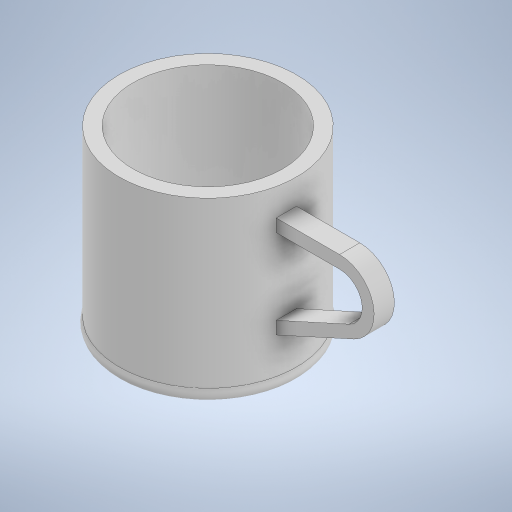
# Autodesk Inventor part: TAZA DEL CID
Saved by Autodesk Inventor 2024 (Build 280153000, 153)
## iProperties
Created: 2024-02-22
Part Number: TAZA DEL CID
Material: Genérico
Document SubType Name: Modeling
Designer: fenyc
Density: 1 g/cm^3
Appearance: Valor por defecto
Author: fenyc
Autodesk Inventor part; units mm, degrees
ref_plane "YZ Plane" through (0, 0, 0) normal (1, 0, 0) x (0, 1, 0)
ref_plane "XZ Plane" through (0, 0, 0) normal (0, 1, 0) x (-1, 0, 0)
ref_plane "XY Plane" through (0, 0, 0) normal (0, 0, 1) x (1, 0, 0)
sketch "Boceto1" plane through (0, 0, 0) normal (0, 0, 1) x (1, 0, 0)
  line L0 (-26.211, 0) -> (6.289, 0)
  line L1 (6.289, 0) -> (6.289, 70)
  line L2 (6.289, 70) -> (-28.711, 70)
  line L3 (-28.711, 70) -> (-28.711, 5)
  arc A0 (-28.711, 5) -> (-26.211, 0) centre (-26.211, 3.125) ccw
  point P0 (0, 0)
  dimension "d2" = 32.5
  dimension "d3" = 70
  dimension "d4" = 35
  dimension "d5" = 65
  constraints: 8 end point, 3 perpendicular, 2 point on circle, 1 centre point, 1 horizontal, 1 tangent
  measures "d2" distance of L0.start L0.end
  measures "d3" distance of L0.end L1.end
  measures "d4" distance of L1.end L2.end
  measures "d5" distance of L2.end L3.end
revolve "Revolución1" add sketch "Boceto1" angle 360 about axis through (6.289, 0, 0) along (0, 1, 0)
sketch "Boceto2" plane through (6.289, 70, 0) normal (0, 1, 0) x (1, 0, 0)
  circle A0 centre (0, 0) radius 29.5174
  point P0 (-6.289, 0)
  constraints: 1 centre point
extrude "Extrusión1" cut sketch "Boceto2" against normal blind 65
sketch "Boceto3" plane through (0, 0, 0) normal (0, 0, 1) x (1, 0, 0)
  line L0 (41.289, 70) -> (-28.711, 70) projected
  line L1 (41.289, 70) -> (41.289, 60)
  line L2 (41.289, 5) -> (41.289, 70) projected
  line L3 (41.289, 60) -> (66.289, 60)
  line L4 (41.289, 5) -> (41.289, 20)
  line L5 (41.289, 20) -> (71.9356, 33.9284)
  arc A0 (71.9356, 33.9284) -> (66.289, 60) centre (66.289, 46.3527) ccw
  line L6 (41.289, 60) -> (41.289, 55)
  line L7 (41.289, 55) -> (66.3769, 55)
  line L8 (41.289, 20) -> (41.289, 25)
  line L9 (41.289, 25) -> (70.0439, 38.0686)
  arc A1 (70.0439, 38.0686) -> (66.3769, 55) centre (66.3769, 46.1372) ccw
  point P0 (0, 0)
  dimension "d9" = 10
  dimension "d10" = 25
  dimension "d11" = 15
  dimension "d12" = 5
  dimension "d13" = 5
  constraints: 16 end point, 4 point on circle, 4 point on line, 4 tangent, 2 centre point, 2 perpendicular, 1 parallel
  measures "d9" distance of L0.start L1.end
  measures "d10" distance of L1.end L3.end
  measures "d11" distance of L2.start L4.end
  measures "d12" distance of L1.end L6.end
  measures "d13" distance of L4.end L8.end
extrude "Extrusión2" add sketch "Boceto3" along normal blind 8 contours L2 L9 A1 L7 L3 A0 L5
